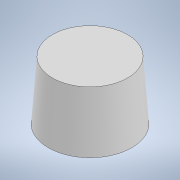
# Autodesk Inventor part: 68. Заглушка
Saved by Autodesk Inventor 2021 (Build 250183000, 183)
## iProperties
Created: 2021-03-11
Part Number: 68. Заглушка
Material: Типовые
Document SubType Name: Modeling
Designer: Данил
Density: 1 g/cm^3
Appearance: По умолчанию
Author: Данил
Autodesk Inventor part; units mm, degrees
ref_plane "YZ Plane" through (0, 0, 0) normal (1, 0, 0) x (0, 1, 0)
ref_plane "XZ Plane" through (0, 0, 0) normal (0, 1, 0) x (-1, 0, 0)
ref_plane "XY Plane" through (0, 0, 0) normal (0, 0, 1) x (1, 0, 0)
sketch "Эскиз1" plane through (0, 0, 0) normal (0, 0, 1) x (1, 0, 0)
  line L0 (0, 3.5) -> (0, -3.5)
  line L1 (0, -3.5) -> (5, -3.5)
  line L2 (5, -3.5) -> (4.5, 3.5)
  line L3 (4.5, 3.5) -> (0, 3.5)
  point P0 (0, 0)
  point P1 (0, 0)
  dimension "d0" = 7
  dimension "d1" = 10
  dimension "d2" = 9
  constraints: 8 end point, 1 coincident, 1 horizontal, 1 midpoint, 1 parallel, 1 vertical
  measures "d0" distance of L0.start L0.end
  measures "d1" diameter of L1.end L0
  measures "d2" diameter of L2.end L0
revolve "Вращение1" add sketch "Эскиз1" angle 360 about axis through (0, 3.5, 0) along (0, -1, 0)
